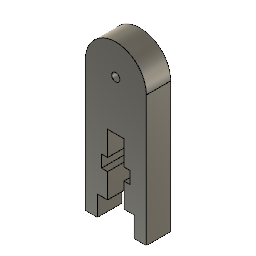
rotor_mount v3 (Autodesk Fusion 360 design; units mm, degrees)
Autodesk Fusion 360 part; units mm, degrees
sketch "Sketch1" plane through (0, 0, 0) normal (0, 1, 0) x (1, 0, 0)
  circle A0 centre (0, 0) radius 28.5
  line L0 (-9, 27.0416) -> (9, 27.0416)
  line L1 (-27.3663, -7.9584) -> (-39.2742, -7.9584)
  line L2 (-49.2742, 2.0416) -> (-49.2742, 27.0416)
  line L3 (-49.2742, 27.0416) -> (-9, 27.0416)
  line L4 (-41.2742, 27.0416) -> (-34.2742, 27.0416)
  line L5 (-34.2742, 27.0416) -> (-34.2742, 2.0416)
  line L6 (-34.2742, 2.0416) -> (-41.2742, 2.0416)
  line L7 (-41.2742, 2.0416) -> (-41.2742, 27.0416)
  line L8 (-41.2742, 2.0416) -> (-49.2742, 2.0416)
  line L9 (-49.2742, 2.0416) -> (-34.2742, 2.0416)
  line L10 (-28.4268, 2.0416) -> (-34.2742, 2.0416)
  line L11 (-44.2742, 11.0416) -> (-31.2742, 11.0416)
  line L12 (-31.2742, 11.0416) -> (-31.2742, 18.0416)
  line L13 (-31.2742, 18.0416) -> (-44.2742, 18.0416)
  line L14 (-44.2742, 18.0416) -> (-44.2742, 11.0416)
  line L15 (-37.7742, 18.0416) -> (-37.7742, 27.0416)
  line L16 (-44.2742, 14.5416) -> (-41.2742, 14.5416)
  line L17 (-44.2742, 11.0416) -> (-49.2742, 11.0416)
  line L18 (-31.2742, 11.0416) -> (-26.2742, 11.0416)
  arc A1 (-49.2742, 2.0416) -> (-39.2742, -7.9584) centre (-39.2742, 2.0416) ccw
  line L19 (0, 27.0416) -> (0, 0)
  line L20 (27.3663, -7.9584) -> (39.2742, -7.9584)
  arc A2 (39.2742, -7.9584) -> (49.2742, 2.0416) centre (39.2742, 2.0416) ccw
  line L21 (49.2742, 2.0416) -> (49.2742, 27.0416)
  line L22 (49.2742, 27.0416) -> (9, 27.0416)
  line L23 (31.2742, 18.0416) -> (44.2742, 18.0416)
  line L24 (31.2742, 11.0416) -> (31.2742, 18.0416)
  line L25 (44.2742, 11.0416) -> (31.2742, 11.0416)
  line L26 (44.2742, 18.0416) -> (44.2742, 11.0416)
  line L27 (41.2742, 2.0416) -> (41.2742, 27.0416)
  line L28 (34.2742, 27.0416) -> (34.2742, 2.0416)
  line L29 (34.2742, 2.0416) -> (41.2742, 2.0416)
  circle A3 centre (0, 0) radius 1
  circle A4 centre (0, 0) radius 7.5
  line L30 (0, 0) -> (-7.5, 0)
  line L31 (-7.5, 0) -> (-7.5, 27.0416)
  line L32 (0, 0) -> (7.5, 0)
  line L33 (7.5, 0) -> (7.5, 27.0416)
  line L34 (-2, 27.0416) -> (2, 27.0416)
  line L35 (2, 27.0416) -> (2, 12.0416)
  line L36 (2, 12.0416) -> (-2, 12.0416)
  line L37 (-2, 12.0416) -> (-2, 27.0416)
  line L38 (-3.5, 18.0416) -> (3.5, 18.0416)
  line L39 (3.5, 18.0416) -> (3.5, 21.0416)
  line L40 (3.5, 21.0416) -> (-3.5, 21.0416)
  line L41 (-3.5, 21.0416) -> (-3.5, 18.0416)
  line L42 (-2, 19.5416) -> (-3.5, 19.5416)
  line L43 (-7.5, 27.0416) -> (-4.5, 27.0416)
  line L44 (-4.5, 27.0416) -> (-4.5, 32.0416)
  line L45 (-4.5, 32.0416) -> (-7.5, 32.0416)
  line L46 (-7.5, 32.0416) -> (-7.5, 27.0416)
  line L47 (7.5, 27.0416) -> (4.5, 27.0416)
  line L48 (4.5, 27.0416) -> (4.5, 32.0416)
  line L49 (4.5, 32.0416) -> (7.5, 32.0416)
  line L50 (7.5, 32.0416) -> (7.5, 27.0416)
  point P0 (0, 21.0416)
  point P1 (0, 27.0416)
  dimension "d1" = 57
  dimension "d2" = 18
  dimension "d3" = 25
  dimension "d4" = 90
  dimension "d5" = 10
  dimension "d8" = 7
  dimension "d9" = 7
  dimension "d10" = 13
  dimension "d11" = 90
  dimension "d12" = 90
  dimension "d13" = 5
  dimension "d14" = 5
  dimension "d15" = 10
  dimension "d18" = 2
  dimension "d19" = 15
  dimension "d20" = 4
  dimension "d21" = 15
  dimension "d22" = 3
  dimension "d23" = 7
  dimension "d24" = 90
  dimension "d25" = 5
  dimension "d26" = 5
  dimension "d27" = 3
  dimension "d28" = 3
  constraint coincident A0.centre L19.end
  constraint coincident A0 L0.start
  constraint coincident A0 L0.end
  constraint horizontal L0
  constraint coincident A0 L1.start
  constraint perpendicular L0 L2
  constraint perpendicular L2 L3
  constraint horizontal L4
  constraint vertical L5
  constraint horizontal L6
  constraint vertical L7
  constraint coincident L3 L4.start
  constraint coincident L2 L8.end
  constraint perpendicular L2 L8
  constraint perpendicular L5 L9
  constraint coincident A0 L10.start
  constraint perpendicular L5 L10
  constraint horizontal L11
  constraint vertical L12
  constraint horizontal L13
  constraint vertical L14
  constraint midpoint L13 L15.start
  constraint midpoint L4 L15.end
  constraint midpoint L14 L16.start
  constraint midpoint L7 L16.end
  constraint perpendicular L2 L17
  constraint coincident A0 L18.end
  constraint perpendicular L12 L18
  constraint coincident L2 L17.end
  constraint tangent L1 A1
  constraint tangent L2 A1
  constraint midpoint L0 P1
  constraint symmetric L0.start L19 L0.end
  constraint symmetric L1.start L19 L20.start
  constraint symmetric L2.end L19 L21.end
  constraint symmetric L4.start L19 L27.end
  constraint symmetric L4.end L19 L28.start
  constraint symmetric L5.end L19 L28.end
  constraint symmetric L6.end L19 L27.start
  constraint symmetric L11.start L19 L25.start
  constraint symmetric L11.end L19 L24.start
  constraint symmetric L12.end L19 L23.start
  constraint symmetric L13.end L19 L23.end
  constraint symmetric L1.end L19 L20.end
  constraint symmetric L2.start L19 A2.end
  constraint symmetric A1 L19 A2
  constraint concentric A3 A4
  constraint coincident A4 L30.end
  constraint perpendicular L19 L30
  constraint coincident L0 L31.end
  constraint tangent A4 L31
  constraint coincident A4 L32.end
  constraint perpendicular L19 L32
  constraint coincident L0 L33.end
  constraint tangent A4 L33
  constraint horizontal L34
  constraint vertical L35
  constraint horizontal L36
  constraint vertical L37
  constraint horizontal L38
  constraint vertical L39
  constraint horizontal L40
  constraint vertical L41
  constraint midpoint L37 L42.start
  constraint midpoint L41 L42.end
  constraint midpoint L40 P0
  constraint midpoint L34 P1
  constraint coincident L19 P0
  constraint coincident P1 L19.start
  constraint horizontal L43
  constraint vertical L44
  constraint horizontal L45
  constraint vertical L46
  constraint horizontal L47
  constraint vertical L48
  constraint horizontal L49
  constraint vertical L50
  measures "d1" diameter of A0
  measures "d2" distance of L0.start L0.end
  measures "d3" distance of L4.end L5.end
  measures "d4" angle of L1 L2
  measures "d5" distance of L1 L6
  measures "d8" distance of L5 L7
  measures "d9" distance of L11.start L13.end
  measures "d10" distance of L12 L14
  measures "d11" angle of L7 L16
  measures "d12" angle of L4 L15
  measures "d13" distance of L11.end L18.end
  measures "d14" distance of L11.start L17.end
  measures "d15" radius of A1
  measures "d18" diameter of A3
  measures "d19" diameter of A4
  measures "d20" distance of L35.end L36.end
  measures "d21" distance of L34.end L35.end
  measures "d22" distance of L38.start L40.end
  measures "d23" distance of L38.start L38.end
  measures "d24" angle of L37 L42
  measures "d25" distance of L31.end L45.end
  measures "d26" distance of L33.end L49.end
  measures "d27" distance of L48.end L49.end
  measures "d28" distance of L44.end L45.end
extrude "Extrude1" add sketch "Sketch1" along normal blind 100 contours A0 L0 L47 L48 L50 | A0 L48 L49 L50 | L0 L19 A4 L33 L35 L36 L38 L39 L40 L47 | L19 A3 A4 L32 | A3 A4 L30 L32 | A0 L0 L43 L44 L46 | A0 L44 L45 L46 | L0 L19 A4 L31 L36 L37 L38 L40 L41 L43 | L19 A3 A4 L30
sketch "Sketch2" plane through (7.5, 0, 0) normal (1, 0, 0) x (0, 1, 0)
  line L0 (0, 0) -> (0, -32.0416)
  line L1 (0, -32.0416) -> (100, -32.0416)
  line L2 (100, -32.0416) -> (100, 0)
  line L3 (100, 0) -> (0, 0)
  line L4 (5, 16.673) -> (106.6592, 16.673)
  line L5 (106.6592, 16.673) -> (106.6592, -53.0106)
  line L6 (106.6592, -53.0106) -> (5, -53.0106)
  line L7 (5, -53.0106) -> (5, 16.673)
  dimension "d29" = 5
  constraint horizontal L4
  constraint vertical L5
  constraint horizontal L6
  constraint vertical L7
  measures "d29" distance of L0 L7
extrude "Extrude2" cut sketch "Sketch2" against normal blind 100 contours L1 L2 L3 L4 L5 L6 L7 | L1 L2 L3 L7
extrude "Extrude3" add 1 faces at (-3.3745, 0, -4.2745) along direction (0, -1, 0) blind 1
